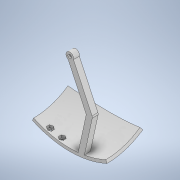
# Autodesk Inventor part: passive_walking_robot5
Saved by Autodesk Inventor 2021 (Build 250183000, 183)
## iProperties
Created: 2024-06-16
Part Number: passive_walking_robot5
Material: 一般
Document SubType Name: Modeling
Designer: 山下　響
Density: 1 g/cm^3
Appearance: 既定
Author: 山下　響
Autodesk Inventor part; units mm, degrees
ref_plane "YZ Plane" through (0, 0, 0) normal (1, 0, 0) x (0, 1, 0)
ref_plane "XZ Plane" through (0, 0, 0) normal (0, 1, 0) x (-1, 0, 0)
ref_plane "XY Plane" through (0, 0, 0) normal (0, 0, 1) x (1, 0, 0)
sketch "スケッチ1" plane through (0, 0, 0) normal (0, 0, 1) x (1, 0, 0)
  arc A0 (-81.314, -122.2088) -> (79.2809, -122.2088) centre (-1.0165, 49.9897) ccw
  line L0 (-1.0165, 49.9897) -> (79.2809, -122.2088) construction
  line L1 (-1.0165, 49.9897) -> (188.9835, 49.9897) construction
  line L2 (-1.0165, 49.9897) -> (-81.314, -122.2088) construction
  arc A1 (-79.2009, -117.6773) -> (77.1678, -117.6773) centre (-1.0165, 49.9897) ccw
  line L3 (-1.0165, 49.9897) -> (77.1678, -117.6773) construction
  line L4 (-1.0165, 49.9897) -> (183.9835, 49.9897) construction
  line L5 (-1.0165, 49.9897) -> (-79.2009, -117.6773) construction
  line L6 (0, -135.0075) -> (35, -74.3858)
  line L7 (0, -135.0075) -> (70, -135.0075) construction
  line L8 (35, -74.3858) -> (2.1456, -4.5601)
  line L9 (35, -74.3858) -> (112.1689, -74.3858) construction
  circle A2 centre (0, 0) radius 2
  circle A3 centre (0, 0) radius 3.075
  circle A4 centre (0, 0) radius 6.5
  line L10 (0, 0) -> (33.3477, -70.8742) construction
  line L11 (-4.5242, -2.1287) -> (28.8235, -73.0029)
  line L12 (37.8719, -68.7455) -> (4.5242, 2.1287)
  arc A5 (4.5242, 2.1287) -> (-4.5242, -2.1287) centre (0, 0) ccw
  arc A6 (28.8235, -73.0029) -> (37.8719, -68.7455) centre (33.3477, -70.8742) ccw
  line L13 (-1.0165, -135.0103) -> (33.3477, -70.8742) construction
  line L14 (3.3907, -137.3717) -> (37.755, -73.2356)
  line L15 (28.9405, -68.5128) -> (-5.4238, -132.6489)
  arc A7 (-5.4238, -132.6489) -> (3.3907, -137.3717) centre (-1.0165, -135.0103) ccw
  arc A8 (37.755, -73.2356) -> (28.9405, -68.5128) centre (33.3477, -70.8742) ccw
  arc A9 (-80.0461, -119.4899) -> (78.0131, -119.4899) centre (-1.0165, 49.9897) ccw
  line L16 (-1.0165, 49.9897) -> (78.0131, -119.4899) construction
  line L17 (-1.0165, 49.9897) -> (185.9835, 49.9897) construction
  line L18 (-1.0165, 49.9897) -> (-80.0461, -119.4899) construction
  line L19 (0, 0) -> (19.103, -135.9248)
  line L20 (0, 0) -> (137.2607, 0) construction
  line L21 (33.3477, -70.8742) -> (19.103, -135.9248) construction
  line L22 (28.4635, -69.8046) -> (14.2187, -134.8553)
  line L23 (23.9873, -136.9944) -> (38.232, -71.9437)
  arc A10 (38.232, -71.9437) -> (28.4635, -69.8046) centre (33.3477, -70.8742) ccw
  arc A11 (14.2187, -134.8553) -> (23.9873, -136.9944) centre (19.103, -135.9248) ccw
  point P0 (0, 0)
  point P1 (16.6739, -35.4371)
  point P2 (16.1656, -102.9423)
  point P3 (6.2925, -1.6294)
  point P4 (-2.756, -5.8868)
  point P5 (27.7533, -70.7285)
  point P6 (37.8719, -68.7455)
  point P7 (-5.6235, -136.9536)
  point P8 (3.6151, -136.953)
  point P9 (37.755, -73.2356)
  point P10 (37.8719, -68.7455)
  point P11 (33.3512, -133.8251)
  point P12 (26.2254, -103.3995)
  point P13 (28.0999, -71.465)
  point P14 (14.1253, -136.3963)
  point P15 (24.3626, -135.2801)
  dimension "d0" = 50
  dimension "d1" = 190
  dimension "d2" = 65
  dimension "d3" = 50
  dimension "d4" = 185
  dimension "d5" = 65
  dimension "d6" = 50
  dimension "d7" = 70
  dimension "d8" = 60
  dimension "d9" = 0
  dimension "d11" = 4
  dimension "d12" = 6.15
  dimension "d13" = 13
  dimension "d14" = 10
  dimension "d15" = 10
  dimension "d16" = 187
  dimension "d17" = 65
  dimension "d18" = 50
  dimension "d34" = 0
  dimension "d35" = 0
  dimension "d36" = 82
  dimension "d37" = 10
  constraints: 54 end point, 22 point on circle, 12 centre point, 12 tangent, 6 equal length, 6 horizontal, 5 coincident, 3 midpoint, 3 parallel, 2 point on line
  measures "d0" distance of point (0, 0) point (-1.017, 49.99)
  measures "d1" radius of A0
  measures "d2" angle of L0 L1
  measures "d3" angle of L2 L0
  measures "d4" radius of A1
  measures "d5" angle of L3 L4
  measures "d6" angle of L5 L3
  measures "d7" distance of L6.start L6.end
  measures "d8" angle of L7 L6
  measures "d9" horizontal distance of point (0, 0) L6.start
  measures "d11" diameter of A2
  measures "d12" diameter of A3
  measures "d13" diameter of A4
  measures "d14" diameter of A6
  measures "d15" diameter of A8
  measures "d16" radius of A9
  measures "d17" angle of L16 L17
  measures "d18" angle of L18 L16
  measures "d34" distance of point (0, 0) A2.centre
  measures "d35" distance of point (0, 0) A2.centre
  measures "d36" angle of L19 L20
  measures "d37" diameter of A11
extrude "押し出し1" add sketch "スケッチ1" along normal mid plane 5 contours A3
extrude "押し出し2" add sketch "スケッチ1" along normal mid plane 10 contours L11 L19 A4 L8 A8 L15 | L11 A4 L19 | L11 A5 L12 A4 | A4 L12 A5 L11 | A8 L8 A4 L12
extrude "押し出し3" add sketch "スケッチ1" along normal mid plane 10 contours A11 L22 A1 L19 A9 | L19 A1 L23 A9 | L19 L22 L14 A6 L23 A1 | A1 L22 L19 | L22 L11 A6 L6 | L6 A6 L14 L22 | L15 A10 L22 L11 | A6 L6 L8 A8 | A6 L11 L22 A10 A8 L8 L6
sketch "スケッチ2" plane through (0, 0, 5) normal (0, 0, 1) x (1, 0, 0)
  line L0 (-17.1369, -20) -> (12.9571, -20)
  arc A0 (-63.3927, -125.9462) -> (63.3927, -125.9462) centre (0, 10) ccw
  line L1 (0, 10) -> (63.3927, -125.9462) construction
  line L2 (0, 10) -> (150, 10) construction
  line L3 (0, 10) -> (-63.3927, -125.9462) construction
  arc A1 (-61.2796, -121.4146) -> (61.2796, -121.4146) centre (0, 10) ccw
  line L4 (0, 10) -> (61.2796, -121.4146) construction
  line L5 (0, 10) -> (145, 10) construction
  line L6 (0, 10) -> (-61.2796, -121.4146) construction
  line L7 (-63.3927, -125.9462) -> (-61.2796, -121.4146)
  line L8 (63.3927, -125.9462) -> (61.2796, -121.4146)
  point P0 (0, 0)
  point P1 (0, -20)
  dimension "d25" = 20
  dimension "d26" = 10
  dimension "d27" = 150
  dimension "d28" = 65
  dimension "d29" = 50
  dimension "d30" = 145
  dimension "d31" = 65
  dimension "d32" = 50
  constraints: 18 end point, 4 point on circle, 3 horizontal, 2 centre point, 2 coincident, 2 equal length
  measures "d25" distance of point (0, 0) point (0, -20)
  measures "d26" distance of point (0, 0) point (0, 10)
  measures "d27" radius of A0
  measures "d28" angle of L1 L2
  measures "d29" angle of L3 L1
  measures "d30" radius of A1
  measures "d31" angle of L4 L5
  measures "d32" angle of L6 L4
revolve "回転1" add sketch "スケッチ2" angle 35 about axis through (-17.1369, -20, 5) along (1, 0, 0)
sketch "スケッチ3" plane through (0, 0, 0) normal (0, 1, 0) x (-1, 0, 0)
  line L0 (-14.3428, 5) -> (61.2796, 5) projected
  circle A0 centre (20, -2) radius 2.5
  line L1 (20, 3) -> (24.3301, 0.5)
  line L2 (24.3301, 0.5) -> (24.3301, -4.5)
  line L3 (24.3301, -4.5) -> (20, -7)
  line L4 (20, -7) -> (15.6699, -4.5)
  line L5 (15.6699, -4.5) -> (15.6699, 0.5)
  line L6 (15.6699, 0.5) -> (20, 3)
  circle A1 centre (40, -2) radius 2.5
  line L7 (40, 3) -> (35.6699, 0.5)
  line L8 (35.6699, 0.5) -> (35.6699, -4.5)
  line L9 (35.6699, -4.5) -> (40, -7)
  line L10 (40, -7) -> (44.3301, -4.5)
  line L11 (44.3301, -4.5) -> (44.3301, 0.5)
  line L12 (44.3301, 0.5) -> (40, 3)
  point P0 (0, 0)
  dimension "d38" = 7
  dimension "d39" = 20
  dimension "d40" = 5
  dimension "d41" = 10
  constraints: 24 end point, 2 centre point, 2 coincident, 13 other
  measures "d38" distance from line of L0 point (20, -2)
  measures "d39" horizontal distance of point (0, 0) point (20, -2)
  measures "d40" diameter of A0
  measures "d41" distance of L3.end L1.start
extrude "押し出し4" cut sketch "スケッチ3" against normal blind 1000 contours A0 | A1
extrude "押し出し5" cut sketch "スケッチ3" against normal blind 132 contours L12 L11 L10 L9 L8 L7
extrude "押し出し6" cut sketch "スケッチ3" against normal blind 137 contours L1 L2 L3 L4 L5 L6
